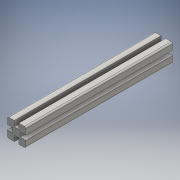
# Autodesk Inventor part: column
Saved by Autodesk Inventor 2016 (Build 200138000, 138)
## iProperties
Created: 2015-09-03
Part Number: column
Material: Generic
Document SubType Name: Modeling
Designer: oscar
Density: 1 g/cm^3
Appearance: Default
Author: oscar
Autodesk Inventor part; units mm, degrees
ref_plane "YZ Plane" through (0, 0, 0) normal (1, 0, 0) x (0, 1, 0)
ref_plane "XZ Plane" through (0, 0, 0) normal (0, 1, 0) x (-1, 0, 0)
ref_plane "XY Plane" through (0, 0, 0) normal (0, 0, 1) x (1, 0, 0)
sketch "Sketch1" plane through (0, 0, 0) normal (0, 1, 0) x (-1, 0, 0)
  line L0 (-5, 20) -> (-5, 8)
  line L1 (5, -20) -> (5, -8)
  line L2 (20, 5) -> (8, 5)
  line L3 (-20, -5) -> (-8, -5)
  line L4 (8, -5) -> (20, -5)
  line L5 (-8, 5) -> (-20, 5)
  line L6 (-5, -8) -> (-5, -20)
  line L7 (5, 8) -> (5, 20)
  arc A0 (-17, 20) -> (-20, 17) centre (-17, 17) ccw
  arc A1 (-20, -17) -> (-17, -20) centre (-17, -17) ccw
  arc A2 (17, -20) -> (20, -17) centre (17, -17) ccw
  arc A3 (20, 17) -> (17, 20) centre (17, 17) ccw
  line L8 (20, 17) -> (20, 5)
  line L9 (20, -5) -> (20, -17)
  line L10 (17, -20) -> (5, -20)
  line L11 (-5, -20) -> (-17, -20)
  line L12 (-20, -17) -> (-20, -5)
  line L13 (-20, 5) -> (-20, 17)
  line L14 (-17, 20) -> (-5, 20)
  line L15 (17, 20) -> (5, 20)
  line L16 (5, 8) -> (-5, 8)
  line L17 (-8, 5) -> (-8, -5)
  line L18 (-5, -8) -> (5, -8)
  line L19 (8, -5) -> (8, 5)
  point P0 (0, 0)
  constraints: 40 end point, 8 point on circle, 6 perpendicular, 4 centre point, 4 collinear, 1 parallel, 1 tangent, 1 vertical
extrude "Extrusion1" add sketch "Sketch1" along normal blind 320
body "Solid1"
